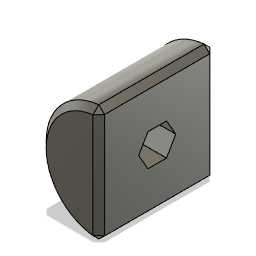
bed center support v2 (Autodesk Fusion 360 design; units mm, degrees)
Autodesk Fusion 360 part; units mm, degrees
sketch "Sketch1" plane through (0, 0, 0) normal (0, 0, 1) x (1, 0, 0)
  line L0 (0, 10) -> (0, -10)
  arc A0 (0, 10) -> (0, -10) centre (0, 0) ccw
  constraint coincident A0.centre origin
  constraint vertical L0
extrude "Extrude1" add sketch "Sketch1" along normal blind 20
sketch "Sketch2" plane through (0, 0, 0) normal (1, 0, 0) x (0, 0, -1)
  line L0 (0, -10) -> (0, 10)
  line L1 (0, 10) -> (-20, 10)
  line L2 (-20, 10) -> (-20, -10)
  line L3 (-20, -10) -> (0, -10)
  line L4 (-8.4123, -2.75) -> (-6.8246, 0)
  line L5 (-6.8246, 0) -> (-8.4123, 2.75)
  line L6 (-8.4123, 2.75) -> (-11.5877, 2.75)
  line L7 (-11.5877, 2.75) -> (-13.1754, 0)
  line L8 (-13.1754, 0) -> (-11.5877, -2.75)
  line L9 (-11.5877, -2.75) -> (-8.4123, -2.75)
  point P0 (-10, 0)
  dimension "d3" = 2.75
  measures "d3" distance of P0 L9
extrude "Extrude2" cut sketch "Sketch2" against normal blind 7 contours L4 L5 L6 L7 L8 L9
chamfer "Chamfer1" distance 1 angle 45 6 edges at (0, 0, 20) (0, 10, 10) (0, -10, 10) (0, 0, 0) (-10, 0, 0) (-10, 0, 20)
equation "d3 = ( 5.5 / 2 ) * 1 mm"
named bodies: "bed center support"
